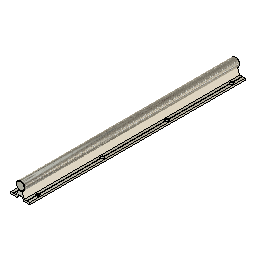
_SBR20 Linear Rail 500 mm v7.6b91af5f-68bf-4e04-9d78-1c30a96e3cb4 (Autodesk Fusion 360 design; units mm, degrees)
Autodesk Fusion 360 part; units mm, degrees
note: some values were not read from the file. Set by a fixed rule: which sketch regions a step uses.
sketch "Sketch1" plane through (0, 0, 0) normal (0, 1, 0) x (1, 0, 0)
  circle A0 centre (0, 0) radius 10
  line L0 (-3.8, 9.2499) -> (-9.425, 22.1)
  line L1 (-9.425, 22.1) -> (-21.925, 22.1)
  line L2 (-21.925, 22.1) -> (-21.925, 26.8)
  line L3 (21.925, 26.8) -> (21.925, 22.1)
  line L4 (21.925, 22.1) -> (9.425, 22.1)
  line L5 (9.425, 22.1) -> (3.8, 9.2499)
  line L6 (0, 26.8) -> (0, 20.3) construction
  line L7 (-21.925, 26.8) -> (-7.925, 26.8)
  line L8 (7.925, 26.8) -> (21.925, 26.8)
  line L9 (-7.925, 26.8) -> (7.925, 26.8) construction
  line L10 (0, 0) -> (0, -10) construction
  line L11 (0, 20.3) -> (4.5, 20.3)
  line L12 (0, 20.3) -> (-4.5, 20.3)
  line L13 (-7.925, 26.8) -> (-4.5, 20.3)
  line L14 (7.925, 26.8) -> (4.5, 20.3)
  line L15 (0, 0) -> (0, 10) construction
  line L16 (0, 10) -> (0, 10.811) construction
  line L17 (0, 10.811) -> (-3.8, 9.2499)
  line L18 (0, 10.811) -> (3.8, 9.2499)
  line L19 (-3.8, 9.2499) -> (0, 9.2499) construction
  line L20 (3.8, 9.2499) -> (0, 9.2499) construction
  line L21 (0, 20.3) -> (0, 10.811) construction
  line L22 (15.675, 22.1) -> (15.675, 22.6) construction
  line L23 (0, 20.3) -> (0, 19.8) construction
  line L24 (-15.675, 22.1) -> (-15.675, 22.6) construction
  line L25 (16.175, 22.1) -> (15.675, 22.6)
  line L26 (15.675, 22.6) -> (15.175, 22.1)
  line L27 (0.5, 20.3) -> (0, 19.8)
  line L28 (0, 19.8) -> (-0.5, 20.3)
  line L29 (-15.175, 22.1) -> (-15.675, 22.6)
  line L30 (-15.675, 22.6) -> (-16.175, 22.1)
  line L31 (15.675, 26.3) -> (15.175, 26.8)
  line L32 (15.675, 26.3) -> (16.175, 26.8)
  line L33 (-15.675, 26.3) -> (-15.175, 26.8)
  line L34 (-15.675, 26.3) -> (-16.175, 26.8)
  line L35 (-15.675, 22.6) -> (-15.675, 26.3) construction
  line L36 (15.675, 22.6) -> (15.675, 26.3) construction
  dimension "d1" = 20
  dimension "d3" = 12.5
  dimension "d4" = 43.85
  dimension "d7" = 4.7
  dimension "d8" = 6.5
  dimension "d10" = 36.8
  dimension "d11" = 14
  dimension "d12" = 4.5
  dimension "d67" = 0.5
  dimension "d68" = 0.5
  dimension "d69" = 0.5
  dimension "d73" = 7.6
  constraint coincident A0.centre L10.start
  constraint coincident A0 L0.start
  constraint perpendicular L1 L2
  constraint perpendicular L3 L7
  constraint equal L0 L5
  constraint equal L1 L4
  constraint equal L2 L3
  constraint perpendicular L6 L7
  constraint coincident L8.start L7
  constraint collinear L7 L8
  constraint coincident L6.start L7
  constraint equal L7 L8
  constraint coincident A0 L10.end
  constraint horizontal L1
  constraint perpendicular L6 L11
  constraint perpendicular L6 L12
  constraint equal L11 L12
  constraint equal L13 L14
  constraint coincident A0 L15.end
  constraint vertical L15
  constraint vertical L10
  constraint equal L17 L18
  constraint tangent A0 L18
  constraint tangent A0 L17
  constraint coincident L15 L19.end
  constraint perpendicular L15 L19
  constraint horizontal L4
  constraint perpendicular L11 L21
  constraint vertical L21
  constraint vertical L16
  constraint midpoint L4 L22.start
  constraint perpendicular L4 L22
  constraint perpendicular L12 L23
  constraint midpoint L1 L24.start
  constraint perpendicular L1 L24
  constraint coincident L4 L25.start
  constraint coincident L4 L26.end
  constraint coincident L11 L27.start
  constraint coincident L12 L28.end
  constraint coincident L1 L29.start
  constraint coincident L1 L30.end
  constraint parallel L27 L30
  constraint equal L29 L30
  constraint equal L28 L29
  constraint equal L26 L27
  constraint equal L25 L26
  constraint perpendicular L25 L26
  constraint coincident L8 L31.end
  constraint coincident L8 L32.end
  constraint coincident L7 L33.end
  constraint coincident L7 L34.end
  constraint parallel L31 L34
  constraint equal L30 L34
  constraint equal L33 L34
  constraint equal L32 L33
  constraint vertical L36
  constraint vertical L35
  constraint equal L35 L36
  measures "d1" diameter of A0
  measures "d3" distance of L0.end L1.end
  measures "d4" distance of L2.end L3.start
  measures "d7" distance of L3.start L3.end
  measures "d8" distance of L6.start L6.end
  measures "d10" vertical distance of L6.start L10.end
  measures "d11" distance of L3.start L8.start
  measures "d12" distance of L6.end L12.end
  measures "d67" distance of L22.start L22.end
  measures "d68" distance of L6.end L23.end
  measures "d69" distance of L24.start L24.end
  measures "d73" distance of L0.start L5.end
extrude "Extrude1" add sketch "Sketch1" along normal blind 500 contours L0 L1 L2 L3 L4 L5 L7 L8 L11 L12 L13 L14 L17 L18 L25 L26 L27 L28 L29 L30 L31 L32 L33 L34 makes body 1
copy_body "Body->Comp1" bodies 1 removing the originals makes body 2 in component "Component"
extrude "Extrude1'" add sketch "Sketch1" along normal blind 500 separate body contours A0 makes body 3 in component "Component'"
chamfer "Chamfer1" distance 1 angle 45 2 edges at (-9.3233, 0, 3.6162) (-9.3233, 500, 3.6162) on bodies 3 in component "Component'"
sketch "Sketch3" plane through (0, 0, -22.1) normal (0, 0, 1) x (-1, 0, 0)
  line L0 (-16.175, 0) -> (-21.925, 0)
  line L1 (-21.925, 0) -> (-21.925, -500)
  line L2 (-21.925, -500) -> (-16.175, -500)
  line L3 (-16.175, -500) -> (-16.175, 0)
  line L4 (15.675, 0) -> (15.675, -500)
  line L5 (-15.675, 0) -> (-15.675, -500)
  line L6 (-15.675, 0) -> (-15.675, -25) construction
  line L7 (-15.675, -25) -> (-15.675, -175) construction
  line L8 (-15.675, -175) -> (-15.675, -325) construction
  line L9 (-15.675, -325) -> (-15.675, -475) construction
  line L10 (-15.675, -475) -> (15.675, -475) construction
  line L11 (-15.675, -325) -> (15.675, -325) construction
  line L12 (-15.675, -175) -> (15.675, -175) construction
  line L13 (-15.675, -25) -> (15.675, -25) construction
  circle A0 centre (15.675, -475) radius 3.135
  circle A1 centre (-15.675, -475) radius 3.135
  circle A2 centre (-15.675, -325) radius 3.135
  circle A3 centre (15.675, -325) radius 3.135
  circle A4 centre (15.675, -175) radius 3.135
  circle A5 centre (-15.675, -175) radius 3.135
  circle A6 centre (15.675, -25) radius 3.135
  circle A7 centre (-15.675, -25) radius 3.135
  circle A8 centre (0, -325) radius 3.135
  circle A9 centre (0, -25) radius 3.135
  circle A10 centre (0, -175) radius 3.135
  circle A11 centre (0, -475) radius 3.135
  dimension "d74" = 25
  dimension "d75" = 150
  dimension "d76" = 150
  dimension "d77" = 150
  dimension "d78" = 6.27
  constraint coincident L5.start L6.start
  constraint perpendicular L0 L6
  constraint parallel L5 L7
  constraint parallel L5 L8
  constraint parallel L5 L9
  constraint coincident L4 L10.end
  constraint perpendicular L4 L10
  constraint coincident L4 L11.end
  constraint perpendicular L4 L11
  constraint coincident L4 L12.end
  constraint perpendicular L4 L12
  constraint coincident L4 L13.end
  constraint perpendicular L4 L13
  constraint coincident L10.end A0.centre
  constraint coincident L9.end L10.start
  constraint coincident L8.end L9.start
  constraint coincident L11.end A3.centre
  constraint coincident L12.end A4.centre
  constraint coincident L7.end L8.start
  constraint coincident L13.end A6.centre
  constraint coincident L6.end L7.start
  constraint equal A6 A7
  constraint equal A5 A7
  constraint equal A4 A5
  constraint equal A3 A4
  constraint equal A2 A3
  constraint equal A1 A2
  constraint equal A0 A1
  constraint midpoint L11 A8.centre
  constraint midpoint L13 A9.centre
  constraint midpoint L12 A10.centre
  constraint midpoint L10 A11.centre
  constraint equal A0 A11
  constraint equal A8 A11
  constraint equal A8 A10
  constraint equal A9 A10
  measures "d74" distance of L5.start L6.end
  measures "d75" distance of L6.end L7.end
  measures "d76" distance of L7.end L8.end
  measures "d77" distance of L8.end L9.end
  measures "d78" diameter of A3
hole "Hole1" at (-15.675, 25, -22.1) at (15.675, 25, -22.1) at (15.675, 175, -22.1) at (-15.675, 175, -22.1) at (15.675, 325, -22.1) at (-15.675, 325, -22.1) at (15.675, 475, -22.1) at (-15.675, 475, -22.1) direction (0, 0, -1) diameter 3.9 depth 5 tip angle 118 countersink diameter 8.2 countersink angle 90 bodies 2 in component "Component"
extrude "Extrude1''" cut sketch "Sketch3" along normal mid plane 27.4421 contours L3 L5 A7 | L3 A7 | L5 A7 | L3 L5 A5 | L3 A5 | L3 A1 | L3 L5 A1 | L5 A5 | L5 A1 | L3 L5 A2 | L3 A2 | L5 A2 | L4 A6 | L4 A6 | L4 A4 | L4 A4 | L4 A3 | L4 A3 | L4 A0 | L4 A0 | A8 | A9 | A10 | A11 bodies 2 in component "Component"
component "Component'" placed x (1, 0, 0) y (0, 1, 0) z (0, 0, 1) at (0, 0, 0)
component "Component" placed x (1, 0, 0) y (0, 1, 0) z (0, 0, 1) at (0, 0, 0)
